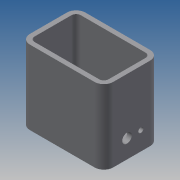
# Autodesk Inventor part: pullbox
Saved by Autodesk Inventor 2014 SP1 (Build 180222100, 222)
## iProperties
Created: 2014-12-12
Part Number: pullbox
Material: Generic
Document SubType Name: Modeling
Designer: Dave
Density: 1 g/cm^3
Appearance: Default
Author: Dave
Autodesk Inventor part; units mm, degrees
ref_plane "YZ Plane" through (0, 0, 0) normal (1, 0, 0) x (0, 1, 0)
ref_plane "XZ Plane" through (0, 0, 0) normal (0, 1, 0) x (-1, 0, 0)
ref_plane "XY Plane" through (0, 0, 0) normal (0, 0, 1) x (1, 0, 0)
sketch "Sketch1" plane through (0, 0, 0) normal (0, 1, 0) x (-1, 0, 0)
  line L0 (101.6, 0) -> (812.8, 0)
  line L1 (914.4, 101.6) -> (914.4, 508)
  line L2 (812.8, 609.6) -> (101.6, 609.6)
  line L3 (0, 508) -> (0, 101.6)
  arc A0 (101.6, 609.6) -> (0, 508) centre (101.6, 508) ccw
  arc A1 (0, 101.6) -> (101.6, 0) centre (101.6, 101.6) ccw
  arc A2 (812.8, 0) -> (914.4, 101.6) centre (812.8, 101.6) ccw
  arc A3 (914.4, 508) -> (812.8, 609.6) centre (812.8, 508) ccw
  point P0 (0, 0)
  point P1 (914.4, 609.6)
  point P2 (914.4, 0)
  point P3 (0, 609.6)
  dimension "d0" = 914.4
  dimension "d1" = 609.6
  dimension "d9" = 101.6
  constraints: 8 end point, 8 point on circle, 8 point on line, 8 tangent, 4 centre point, 3 equal radius, 2 parallel, 1 horizontal, 1 perpendicular
  measures "d0" distance of point (0, 609.6) point (914.4, 609.6)
  measures "d1" distance of point (914.4, 609.6) point (914.4, 0)
  measures "d9" radius of A0
extrude "Extrusion1" add sketch "Sketch1" along normal blind 50.8
sketch "Sketch3" plane through (0, 50.8, 0) normal (0, 1, 0) x (1, 0, 0)
  line L0 (0, -508) -> (0, -101.6) projected
  arc A0 (0, -101.6) -> (-101.6, 0) centre (-101.6, -101.6) ccw projected
  line L1 (-101.6, 0) -> (-812.8, 0) projected
  arc A1 (-812.8, 0) -> (-914.4, -101.6) centre (-812.8, -101.6) ccw projected
  line L2 (-914.4, -101.6) -> (-914.4, -508) projected
  arc A2 (-914.4, -508) -> (-812.8, -609.6) centre (-812.8, -508) ccw projected
  line L3 (-812.8, -609.6) -> (-101.6, -609.6) projected
  arc A3 (-101.6, -609.6) -> (0, -508) centre (-101.6, -508) ccw projected
  line L4 (-812.8, -50.8) -> (-101.6, -50.8)
  arc A4 (-50.8, -101.6) -> (-101.6, -50.8) centre (-101.6, -101.6) ccw
  line L5 (-50.8, -101.6) -> (-50.8, -508)
  arc A5 (-101.6, -558.8) -> (-50.8, -508) centre (-101.6, -508) ccw
  line L6 (-101.6, -558.8) -> (-812.8, -558.8)
  arc A6 (-863.6, -508) -> (-812.8, -558.8) centre (-812.8, -508) ccw
  line L7 (-863.6, -508) -> (-863.6, -101.6)
  arc A7 (-812.8, -50.8) -> (-863.6, -101.6) centre (-812.8, -101.6) ccw
  point P0 (0, 0)
  dimension "d10" = 50.8
  constraints: 8 end point, 8 point on circle, 4 centre point, 7 other
  measures "d10" distance between parallel lines of L4 L1
extrude "Extrusion3" add sketch "Sketch3" along normal blind 762
sketch "Sketch6" plane through (0, 0, 508) normal (1, 0, 0) x (0, 0, -1)
  line L0 (0, 812.8) -> (406.4, 812.8) projected
  line L1 (0, 0) -> (0, 812.8) projected
  circle A0 centre (152.4, 203.2) radius 21.7288
  point P0 (508, 0)
  dimension "d35" = 609.6
  dimension "d36" = 152.4
  constraints: 1 centre point
  measures "d35" distance from line of A0.centre L0
  measures "d36" distance from line of L1 A0.centre
hole "Hole3" at (0, 203.2, 355.6) direction (-1, 0, 0) diameter 105 end through all
sketch "Sketch7" plane through (0, 0, 508) normal (1, 0, 0) x (0, 0, -1)
  circle A0 centre (152.4, 203.2) radius 52.5 projected
  circle A1 centre (304.8, 203.2) radius 31.75
  point P0 (508, 0)
  dimension "d44" = 63.5
  dimension "d45" = 152.4
  constraints: 1 centre point
  measures "d44" diameter of A1
  measures "d45" distance of A1.centre A0.centre
hole "Hole4" at (0, 203.2, 203.2) direction (-1, 0, 0) diameter 55 depth 152.4 tip angle 118
body "Solid1"
